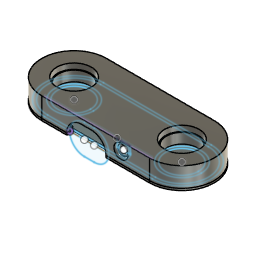
2025_10_24_OdileFootBoardOneFoot v5 (Autodesk Fusion 360 design; units mm, degrees)
Autodesk Fusion 360 part; units mm, degrees
sketch "Sketch1" plane through (0, 0, 0) normal (0, 0, 1) x (1, 0, 0)
  line L0 (0, 0) -> (40, 0)
  line L1 (40, 0) -> (40, 60)
  line L2 (40, 60) -> (0, 60)
  line L3 (0, 60) -> (0, 0)
  line L4 (40, 60) -> (39, 60) construction
  line L5 (39, 60) -> (39, 59) construction
  line L6 (39, 59) -> (40, 59) construction
  line L7 (40, 59) -> (40, 60) construction
  line L8 (0, 60) -> (1, 60) construction
  line L9 (1, 60) -> (1, 59) construction
  line L10 (1, 59) -> (0, 59) construction
  line L11 (0, 59) -> (0, 60) construction
  line L12 (0, 0) -> (1, 0) construction
  line L13 (1, 0) -> (1, 1) construction
  line L14 (1, 1) -> (0, 1) construction
  line L15 (0, 1) -> (0, 0) construction
  line L16 (40, 0) -> (39, 0) construction
  line L17 (39, 0) -> (39, 1) construction
  line L18 (39, 1) -> (40, 1) construction
  line L19 (40, 1) -> (40, 0) construction
  line L20 (39, 1) -> (38, 1)
  line L21 (38, 1) -> (38, 2)
  line L22 (38, 2) -> (39, 2)
  line L23 (39, 2) -> (39, 1)
  line L24 (1, 1) -> (2, 1)
  line L25 (2, 1) -> (2, 2)
  line L26 (2, 2) -> (1, 2)
  line L27 (1, 2) -> (1, 1)
  line L28 (39, 59) -> (38, 59)
  line L29 (38, 59) -> (38, 58)
  line L30 (38, 58) -> (39, 58)
  line L31 (39, 58) -> (39, 59)
  line L32 (1, 59) -> (2, 59)
  line L33 (2, 59) -> (2, 58)
  line L34 (2, 58) -> (1, 58)
  line L35 (1, 58) -> (1, 59)
  dimension "d1" = 40
  dimension "d2" = 60
  dimension "d3" = 1
  dimension "d4" = 1
  dimension "d5" = 1
  dimension "d6" = 1
  dimension "d7" = 1
  dimension "d8" = 1
  dimension "d9" = 1
  dimension "d10" = 1
  dimension "d11" = 1
  dimension "d12" = 1
  dimension "d13" = 1
  dimension "d14" = 1
  dimension "d15" = 1
  dimension "d16" = 1
  dimension "d17" = 1
  dimension "d18" = 1
  constraint horizontal L0
  constraint vertical L1
  constraint horizontal L2
  constraint vertical L3
  constraint coincident L0.start L3.end
  constraint horizontal L4
  constraint vertical L5
  constraint horizontal L6
  constraint vertical L7
  constraint horizontal L8
  constraint vertical L9
  constraint horizontal L10
  constraint vertical L11
  constraint horizontal L12
  constraint vertical L13
  constraint horizontal L14
  constraint vertical L15
  constraint horizontal L16
  constraint vertical L17
  constraint horizontal L18
  constraint vertical L19
  constraint horizontal L20
  constraint vertical L21
  constraint horizontal L22
  constraint vertical L23
  constraint horizontal L24
  constraint vertical L25
  constraint horizontal L26
  constraint vertical L27
  constraint horizontal L28
  constraint vertical L29
  constraint horizontal L30
  constraint vertical L31
  constraint horizontal L32
  constraint vertical L33
  constraint horizontal L34
  constraint vertical L35
  measures "d1" distance of L0.start L0.end
  measures "d2" distance of L0.start L2.end
  measures "d3" distance of L1.end L4.end
  measures "d4" distance of L1.end L6.end
  measures "d5" distance of L2.end L8.end
  measures "d6" distance of L2.end L10.end
  measures "d7" distance of L0.start L12.end
  measures "d8" distance of L0.start L14.end
  measures "d9" distance of L0.end L16.end
  measures "d10" distance of L0.end L18.end
  measures "d11" distance of L17.end L20.end
  measures "d12" distance of L17.end L22.end
  measures "d13" distance of L13.end L24.end
  measures "d14" distance of L13.end L26.end
  measures "d15" distance of L5.end L28.end
  measures "d16" distance of L5.end L30.end
  measures "d17" distance of L9.end L32.end
  measures "d18" distance of L9.end L34.end
sketch "Sketch2" plane through (0, 0, 0) normal (0, 0, 1) x (1, 0, 0)
  circle A0 centre (-25.5102, 30) radius 15
  circle A1 centre (-25.5102, 30) radius 16.75
  line L0 (40, 0) -> (40, 60)
  line L1 (14.4898, 30) -> (84.4898, 30) construction
  line L2 (40, 60) -> (0, 60) construction
  line L3 (14.4898, 30) -> (-25.5102, 30) construction
  circle A2 centre (84.4898, 30) radius 15
  circle A3 centre (84.4898, 30) radius 16.75
  line L4 (84.4898, 60) -> (-25.5102, 60)
  arc A4 (-25.5102, 60) -> (-25.5102, 0) centre (-25.5102, 30) ccw
  line L5 (-25.5102, 0) -> (84.4898, 0)
  arc A5 (84.4898, 0) -> (84.4898, 60) centre (84.4898, 30) ccw
  line L6 (84.4898, 30) -> (-25.5102, 30) construction
  line L7 (84.4898, 63) -> (-25.5102, 63)
  arc A6 (-25.5102, 63) -> (-25.5102, -3) centre (-25.5102, 30) ccw
  line L8 (-25.5102, -3) -> (84.4898, -3)
  arc A7 (84.4898, -3) -> (84.4898, 63) centre (84.4898, 30) ccw
  dimension "d19" = 30
  dimension "d20" = 33.5
  dimension "d21" = 70
  dimension "d22" = 40
  dimension "d23" = 30
  dimension "d24" = 33.5
  dimension "d53" = 3
  constraint concentric A0 A1
  constraint perpendicular L0 L1
  constraint parallel L2 L3
  constraint concentric A2 A3
  constraint coincident L1.end A2.centre
  constraint coincident A0.centre A1.centre
  constraint tangent L4 A4
  constraint tangent A4 L5
  constraint parallel L4 L5
  constraint tangent L5 A5
  constraint tangent L4 A5
  constraint parallel L3 L6
  measures "d19" diameter of A0
  measures "d20" diameter of A1
  measures "d21" distance of L1.start L1.end
  measures "d22" distance of L1.start A0.centre
  measures "d23" diameter of A2
  measures "d24" diameter of A3
sketch "Sketch3" plane through (0, 0, 0) normal (0, 0, 1) x (1, 0, 0)
extrude "Extrude1" add sketch "Sketch1" along normal blind 15 makes body 1
extrude "Extrude2" add sketch "Sketch2" against normal blind 20 separate body contours A0 | A2 makes body 2 at (99.4711, 29.2523, -13.3333) makes body 3 at (-10.5289, 29.2523, -13.3333)
extrude "Extrude3" add sketch "Sketch2" against normal blind 5 contours A1 | A3 bodies 2 3
move_body "Move1" bodies 3 2 to x (1, 0, 0) y (0, 1, 0) z (0, 0, 1) at (0, 0, 20)
extrude "Extrude6" add sketch "Sketch2" along normal blind 20 separate body contours L7 A6 L8 A7 makes body 4
extrude "Extrude4" add sketch "Sketch2" along normal blind 20 separate body contours A0 | A1 | L0 L4 A4 L5 | L0 L4 L5 A5 | A2 | A3 makes body 5
combine "Combine1" operation cut target body 5 tool bodies 2 3
sketch "Sketch4" plane through (0, 0, 0) normal (0, 0, 1) x (1, 0, 0)
  line L0 (84.4898, 60) -> (-25.5102, 60)
  arc A0 (-25.5102, 60) -> (-25.5102, 0) centre (-25.5102, 30) ccw
  line L1 (-25.5102, 0) -> (84.4898, 0)
  arc A1 (84.4898, 0) -> (84.4898, 60) centre (84.4898, 30) ccw
  circle A2 centre (84.4898, 30) radius 16.75
  circle A3 centre (-25.5102, 30) radius 16.75
  line L2 (84.4898, 57) -> (-25.5102, 57)
  arc A4 (-25.5102, 57) -> (-25.5102, 3) centre (-25.5102, 30) ccw
  line L3 (-25.5102, 3) -> (84.4898, 3)
  arc A5 (84.4898, 3) -> (84.4898, 57) centre (84.4898, 30) ccw
  circle A6 centre (-25.5102, 30) radius 19.75
  circle A7 centre (84.4898, 30) radius 19.75
  dimension "d35" = 33.5
  dimension "d36" = 33.5
  dimension "d37" = -3
  dimension "d38" = 3
  dimension "d39" = 3
  constraint tangent L0 A0
  constraint tangent A0 L1
  constraint parallel L0 L1
  constraint tangent L1 A1
  constraint tangent L0 A1
  constraint coincident A0.centre A3.centre
  constraint coincident A1.centre A2.centre
  measures "d35" diameter of A3
  measures "d36" diameter of A2
move_body "Move3" bodies 1 to x (1, 0, 0) y (0, 1, 0) z (0, 0, 1) at (0, 0, 5)
extrude "Extrude5" cut sketch "Sketch4" along normal blind 18 contours L0 A0 L1 A1 | L2 A4 L3 A5 bodies 5
copy_body "CopyPasteBodies1" bodies 1 makes body 6
move_body "Move4" bodies 6 to x (1, 0, 0) y (0, 1, 0) z (0, 0, 1) at (0, 0, 0)
draft "Draft1" angle 10 neutral plane through (0, 0, 15) pull (0, 0, 1) 1 faces at (-8.781, 29.1651, 16.6667) on bodies 5
draft "Draft2" angle 10 neutral plane through (0, 0, 15) pull (0, 0, 1) 1 faces at (101.219, 29.1651, 16.6667) on bodies 5
draft "Draft3" angle -3 neutral plane through (0, 0, 0) pull (0, 0, -1) 1 faces at (99.4152, 28.5065, 5) on bodies 5
draft "Draft4" angle -3 neutral plane through (0, 0, 0) pull (0, 0, -1) 1 faces at (-10.5848, 28.5065, 5) on bodies 5
sketch "Sketch5" plane through (0, 0, 0) normal (0, -1, 0) x (1, 0, 0)
  line L0 (84.4898, 18) -> (84.4898, 20)
  line L1 (84.4898, 20) -> (-25.5102, 20)
  line L2 (-25.5102, 20) -> (-25.5102, 18)
  line L3 (15, -15) -> (25, -15)
  arc A0 (25, -15) -> (25, 15) centre (25, 0) ccw
  line L4 (25, 15) -> (15, 15)
  arc A1 (15, 15) -> (15, -15) centre (15, 0) ccw
  line L5 (0, 0) -> (40, 0) construction
  line L6 (-25.5102, 18) -> (84.4898, 18)
  circle A2 centre (55.2964, 11.2752) radius 5.2
  line L7 (60.3621, 10.1009) -> (50.2308, 10.1009)
  line L8 (62.0719, 10.1009) -> (48.3322, 10.1009)
  line L9 (48.3322, 10.1009) -> (48.3322, 18)
  line L10 (48.3322, 18) -> (62.0719, 18)
  line L11 (62.0719, 18) -> (62.0719, 10.1009)
  circle A3 centre (55.2964, 11.2752) radius 6.8473
  dimension "d70" = 10.4
  constraint tangent L3 A0
  constraint tangent A0 L4
  constraint parallel L3 L4
  constraint tangent L4 A1
  constraint tangent L3 A1
  constraint midpoint A1 L5.start
  constraint midpoint A0 L5.end
  constraint coincident L5.start origin
  constraint coincident A2 L7.start
  constraint coincident A2 L7.end
  constraint horizontal L7
  constraint horizontal L8
  constraint vertical L9
  constraint horizontal L10
  constraint vertical L11
  constraint coincident L6 L9.end
  constraint concentric A2 A3
  measures "d70" diameter of A2
extrude "Extrude7" cut 1 faces at (26, 20.6667, 5) along direction (0, 0, 1) blind 10 on bodies 6 bodies 6
extrude "Extrude8" add 1 faces at (40, 20, 16.6667) along direction (1, 0, 0) blind 4 separate body on bodies 6 makes body 7
extrude "Extrude9" add 1 faces at (0, 40, 16.6667) along direction (-1, 0, 0) blind 4 separate body on bodies 6 makes body 8
delete_body "RemoveBody1" bodies 6
extrude "Extrude10" add 2 faces at (41.3333, 20, 15) (-1.3333, 40, 15) along direction (0, 0, -1) blind 3 on bodies 7 8 bodies 4 5 7 8
extrude "Extrude11" cut sketch "Sketch5" along normal blind 3 contours A2 L7 L8 | A2 L7 L8 bodies 4
extrude "Extrude12" add sketch "Sketch5" against normal blind 19 contours L6 L10 L11 A3 | L6 A2 L8 L10 L11 A3 | L6 L8 L9 L10 A3 | L8 L11 A3 bodies 5 4
fillet "Fillet1" radius 2 1 edges at (50.4483, -3, 13.1556) on bodies 5
extrude "Extrude13" cut sketch "Sketch5" along normal blind 5 contours L3 A0 L4 A1 bodies 5
extrude "Extrude14" cut 2 faces at (-7.4729, 28.2736, 0) (102.5271, 28.2736, 0) along direction (0, 0, 1) blind 5 on bodies 5 bodies 5
draft "Draft5" angle 12 neutral plane through (0, 0, 18) pull (0, 0, -1) 1 faces at (-45.2357, 30.9845, 9.3333) on bodies 5
draft "Draft6" angle 12 neutral plane through (0, 0, 18) pull (0, 0, -1) 1 faces at (64.7643, 30.9845, 9.3333) on bodies 5
sketch "Sketch6" plane through (0, 0, 0) normal (0, 0, -1) x (1, 0, 0)
  line L0 (0, 0) -> (0, 3)
  line L1 (0, 3) -> (-25.5102, 3)
  arc A0 (-25.5102, 3) -> (-25.5102, -63) centre (-25.5102, -30) ccw
  line L2 (-25.5102, -63) -> (84.4898, -63)
  arc A1 (84.4898, -63) -> (84.4898, 3) centre (84.4898, -30) ccw
  line L3 (84.4898, 3) -> (40, 3)
  line L4 (40, 3) -> (40, 0)
  line L5 (40, 0) -> (84.4898, 0)
  arc A2 (84.4898, -60) -> (84.4898, 0) centre (84.4898, -30) ccw
  line L6 (84.4898, -60) -> (-25.5102, -60)
  arc A3 (-25.5102, 0) -> (-25.5102, -60) centre (-25.5102, -30) ccw
  line L7 (-25.5102, 0) -> (0, 0)
extrude "Extrude15" add sketch "Sketch4" along normal blind 20 separate body contours L0 A0 L1 A1 makes body 9
extrude "Extrude16" add sketch "Sketch4" against normal blind 4 contours L0 A0 L1 A1 bodies 9
sketch "Sketch7" plane through (0, 0, 0) normal (0, 0, 1) x (1, 0, 0)
  line L0 (84.4898, 60) -> (-41.8238, 60)
  line L1 (-41.8238, 60) -> (-41.8238, 0)
  line L2 (-41.8238, 0) -> (84.4898, 0)
  line L3 (84.4898, 0) -> (84.4898, 60)
  line L4 (84.4898, 60) -> (101.168, 60)
  line L5 (101.168, 60) -> (101.168, 0)
  line L6 (101.168, 0) -> (84.4898, 0)
  line L7 (84.4898, 0) -> (84.4898, 60)
  point P0 (84.4898, 60)
  constraint horizontal L0
  constraint vertical L1
  constraint horizontal L2
  constraint vertical L3
  constraint coincident P0 L0.start
  constraint horizontal L4
  constraint vertical L5
  constraint horizontal L6
  constraint vertical L7
extrude "Extrude17" cut sketch "Sketch7" along normal blind 35 and the other way blind 10 bodies 9 makes body 10 at (-42.9989, 54.3751, 12)
extrude "Extrude18" cut 2 faces at (113.3699, 32.0233, -4) (-54.3866, 27.9444, -4) along direction (0, 0, 1) blind 6.5 on bodies 9 10 bodies 9 10
draft "Draft7" angle -15 neutral plane through (0, 0, 2.5) pull (0, 0, -1) 1 faces at (-43.7824, 49.8778, 8.3333) on bodies 10
draft "Draft8" angle -15 neutral plane through (0, 0, 2.5) pull (0, 0, -1) 1 faces at (103.0642, 10.4043, 14.1667) on bodies 9
combine "Combine2" operation add target body 5 tool bodies 9 10
extrude "Extrude19" add sketch "Sketch4" 1 faces at (47.8231, 62, 0) along normal blind 2 separate body contours L0 A0 L1 A1 | A2 | A3 | L2 A4 L3 A5 | A6 | A7 on bodies 5 makes body 11
extrude "Extrude20" add sketch "Sketch4" against normal blind 3 contours L0 A0 L1 A1 bodies 11
draft "Draft9" angle -15 neutral plane through (0, 0, -3) pull (0, 0, -1) 4 faces at (32.9932, 0, -2) (-43.6244, 6.086, -1) (47.8231, 60, -2) (96.1428, 57.6443, -2) on bodies 11
mirror "Mirror1" about plane through (0, 0, 2) normal (0, 0, 1) of bodies 11 makes body 12
delete_body "RemoveBody2" bodies 11
move_body "Move5" bodies 12 to x (1, 0, 0) y (0, 1, 0) z (0, 0, 1) at (0, 0, -4)
extrude "Extrude21" cut sketch "Sketch5" against normal blind 4 contours L3 A0 L4 A1 bodies 12
hidden bodies 1
named bodies: "FootBoard", "BottomPart", "BottomPart (1)"
